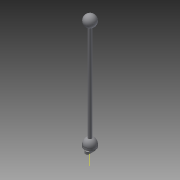
# Autodesk Inventor part: EarShapeET
Saved by Autodesk Inventor 2014 SP1 (Build 180222100, 222)
## iProperties
Created: 2013-10-30
Part Number: EarShapeET
Material: Generic
Document SubType Name: Modeling
Designer: david
Density: 1 g/cm^3
Appearance: Default
Mass: 53.4443 g
Surface Area: 145.67 cm^2
Volume: 53.4443 cm^3
Author: david
Autodesk Inventor part; units mm, degrees
ref_plane "YZ Plane" through (0, 0, 0) normal (1, 0, 0) x (0, 1, 0)
ref_plane "XZ Plane" through (0, 0, 0) normal (0, 1, 0) x (-1, 0, 0)
ref_plane "XY Plane" through (0, 0, 0) normal (0, 0, 1) x (1, 0, 0)
sketch "Sketch1" plane through (0, 0, 0) normal (0, 1, 0) x (-1, 0, 0)
  circle A0 centre (0, 0) radius 5
  dimension "d0" = 10
  constraints: 1 centre point, 1 coincident
  measures "d0" diameter of A0
extrude "Extrusion1" add sketch "Sketch1" along normal blind 2
sketch "Sketch2" plane through (0, 0, 0) normal (0, -1, 0) x (1, 0, 0)
  circle A0 centre (0, 0) radius 5 projected
  circle A1 centre (0, 0) radius 1.5
  dimension "d3" = 3
  constraints: 1 centre point, 1 coincident
  measures "d3" diameter of A1
extrude "Extrusion2" add sketch "Sketch2" along normal blind 2.2 contours A1
sketch "Sketch3" plane through (0, -2.2, 0) normal (0, -1, 0) x (1, 0, 0)
  circle A0 centre (0, 0) radius 1.5 projected
  line L0 (-1.5, 3.4914) -> (-1.5, -3.4914)
  line L1 (1.5, 3.4914) -> (1.5, -3.4914)
  line L2 (0, 15.7328) -> (0, -15.032) construction
  circle A1 centre (0, 0) radius 5 construction
  arc A2 (-2, 4.5826) -> (-2, -4.5826) centre (0, 0) ccw construction
  arc A3 (2, -4.5826) -> (2, 4.5826) centre (0, 0) ccw construction
  arc A4 (1.5, 3.4914) -> (-1.5, 3.4914) centre (0, 0) ccw
  arc A5 (-1.5, -3.4914) -> (1.5, -3.4914) centre (0, 0) ccw
  dimension "d13" = 3.8
  dimension "d19" = 3.8
  constraints: 12 point on circle, 6 end point, 4 centre point, 2 coincident, 2 parallel, 2 tangent, 1 concentric, 1 vertical
  measures "d13" radius of A4
  measures "d19" radius of A5
extrude "Extrusion3" add sketch "Sketch3" along normal blind 1.8
fillet "Fillet2" radius 0.8 4 edges at (-1.5, -3.1, 3.4914) (1.5, -3.1, 3.4914) (-1.5, -3.1, -3.4914) (1.5, -3.1, -3.4914)
ref_plane "Work Plane1" through (0, -2.2, 1.5) normal (1, 0, 0) x (0, 0, -1)
sketch "Sketch8" plane through (0, -2.2, 1.5) normal (1, 0, 0) x (0, 0, -1)
  line L0 (-2.3, -1.8) -> (27.7, -1.8) construction
  line L1 (-62.7924, 4.2) -> (54.2342, 4.2) construction
  line L2 (6.5, 2.2) -> (6.5, -147.8) construction
  arc A0 (6.5, 4.2) -> (3, 8.9697) centre (1.5, 4.2) ccw
  line L3 (-2.3, -1.8) -> (-1.9914, -1.8) projected
  line L4 (3, 8.9697) -> (3, 4.2)
  line L5 (3, 4.2) -> (6.5, 4.2)
  line L6 (-3.5, 2.2) -> (6.5, 2.2) projected
  line L7 (1.5, 2.2) -> (11.5, 2.2) construction
  line L8 (1.5, 4.2) -> (3, 4.2)
  line L9 (3, 4.2) -> (3, 103.9697)
  line L10 (1.5, 104.2) -> (1.5, 4.2)
  line L11 (1.5, 2.2) -> (1.5, 201.2325) construction
  arc A1 (1.5, 94.2) -> (1.5, 104.2) centre (1.5, 99.2) ccw
  line L12 (1.5, 104.2) -> (1.5, 94.2) construction
  line L13 (3, 103.9697) -> (1.5, 104.2)
  line L14 (1.5, 104.2) -> (1.5, 94.2)
  line L15 (1.5, -218.6065) -> (1.5, 270.0391) projected
  point P0 (37.0288, 0)
  point P1 (-2.1951, -1.8)
  dimension "d54" = 30
  dimension "d58" = 6
  dimension "d61" = 150
  dimension "d64" = 0
  dimension "d65" = 1.5
  dimension "d66" = 100
  dimension "d68" = 5
  dimension "d70" = 5
  constraints: 26 end point, 6 collinear, 6 point on line, 5 point on circle, 2 centre point, 2 horizontal, 2 parallel, 1 perpendicular
  measures "d54" distance of L0.start L0.end
  measures "d58" distance between parallel lines of L0 L1
  measures "d61" distance of L2.start L2.end
  measures "d64" distance from line of L3 L0.start
  measures "d65" distance between parallel lines of L9 L10
  measures "d66" distance of L10.start L8.start
  measures "d68" radius of A0
  measures "d70" radius of A1
revolve "Revolution4" add sketch "Sketch8" angle 360 about axis through (0, 2, 0) along (0, 1, 0)
equation "\"d0\" = HeadConnectorOuterSize"
equation "\"d1\" = EarConnectorHeight"
equation "\"d3\" = HeadConnectorWidth - HeadConnectorTolerance"
equation "\"d4\" = HeadConnectorOuterHeight + HeadConnectorTolerance"
equation "\"d13\" = 0.5 * HeadConnectorDiam - HeadConnectorTolerance"
equation "\"d19\" = 0.5 * HeadConnectorDiam - HeadConnectorTolerance"
equation "\"d10\" = HeadConnectorHeight - HeadConnectorTolerance"
equation "\"d20\" = 2 * HeadConnectorProportion"
equation "\"d58\" = HeadConnectorOuterHeight + HeadConnectorHeight + EarConnectorHeight"
equation "\"d65\" = 0.5 * EarWidth"
equation "\"d66\" = EarHeight"
equation "\"d68\" = 0.5 * HeadConnectorOuterSize"
equation "\"d70\" = 0.5 * EarBallSize"
equation "\"EarHeight\" = 100"
equation "\"EarWidth\" = 3"
equation "\"HeadConnectorOuterSize\" = 10"
equation "\"EarConnectorHeight\" = 2"
equation "\"HeadConnectorWidth\" = 3.2"
equation "\"HeadConnectorTolerance\" = 0.2"
equation "\"HeadConnectorOuterHeight\" = 2"
equation "\"HeadConnectorDiam\" = 8"
equation "\"HeadConnectorHeight\" = 2"
equation "\"HeadConnectorProportion\" = 0.4"
equation "\"EarBallSize\" = 10"
body "Solid1"
